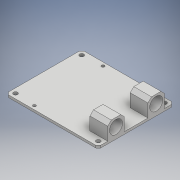
# Autodesk Inventor part: powersupplymount
Saved by Autodesk Inventor 2018.3 (Build 223284000, 284)
## iProperties
Created: 2019-05-29
Part Number: powersupplymount
Material: Generic
Document SubType Name: Modeling
Designer: matth
Density: 1 g/cm^3
Appearance: Default
Author: matth
Autodesk Inventor part; units mm, degrees
ref_plane "YZ Plane" through (0, 0, 0) normal (1, 0, 0) x (0, 1, 0)
ref_plane "XZ Plane" through (0, 0, 0) normal (0, 1, 0) x (-1, 0, 0)
ref_plane "XY Plane" through (0, 0, 0) normal (0, 0, 1) x (1, 0, 0)
sketch "Sketch1" plane through (0, 0, 0) normal (0, 0, 1) x (1, 0, 0)
  line L0 (-9.8382, 8.8164) -> (64.1618, 8.8164)
  line L1 (66.1618, 6.8164) -> (66.1618, -53.1836)
  line L2 (64.1618, -55.1836) -> (-9.8382, -55.1836)
  line L3 (-11.8382, -53.1836) -> (-11.8382, 6.8164)
  line L4 (-9.8382, 8.8164) -> (-11.8382, 6.8164)
  line L5 (64.1618, 8.8164) -> (66.1618, 6.8164)
  line L6 (66.1618, -53.1836) -> (64.1618, -55.1836)
  line L7 (-11.8382, -53.1836) -> (-9.8382, -55.1836)
  circle A0 centre (9.1618, 5.8164) radius 1.25
  circle A1 centre (9.1618, -52.1836) radius 1.25
  circle A2 centre (-7.8382, 4.8164) radius 1.75
  circle A3 centre (-7.8382, -51.1836) radius 1.75
  circle A4 centre (62.1618, -51.1836) radius 1.75
  circle A5 centre (62.1618, 4.8164) radius 1.75
  point P0 (0, 0)
  point P1 (-11.8382, 8.8164)
  point P2 (66.1618, -55.1836)
  point P3 (66.1618, 8.8164)
  point P4 (-11.8382, -55.1836)
  dimension "d0" = 78
  dimension "d1" = 64
  dimension "d2" = 2
  dimension "d3" = 2
  dimension "d4" = 2
  dimension "d5" = 2
  dimension "d6" = 2
  dimension "d7" = 2
  dimension "d8" = 2
  dimension "d9" = 2
  dimension "d10" = 2.5
  dimension "d11" = 21
  dimension "d12" = 3
  dimension "d13" = 2.5
  dimension "d14" = 3
  dimension "d15" = 21
  dimension "d16" = 3.5
  dimension "d17" = 4
  dimension "d18" = 4
  dimension "d19" = 3.5
  dimension "d20" = 4
  dimension "d21" = 4
  dimension "d22" = 3.5
  dimension "d23" = 4
  dimension "d24" = 4
  dimension "d25" = 3.5
  dimension "d26" = 4
  dimension "d27" = 4
  constraints: 16 end point, 8 point on line, 6 centre point, 2 parallel, 1 horizontal, 1 perpendicular
  measures "d0" distance of point (66.162, -55.184) point (-11.838, -55.184)
  measures "d1" distance of point (66.162, 8.816) point (66.162, -55.184)
  measures "d2" distance of L0.start point (-11.838, 8.816)
  measures "d3" distance of L3.end point (-11.838, 8.816)
  measures "d4" distance of L0.end point (66.162, 8.816)
  measures "d5" distance of L1.start point (66.162, 8.816)
  measures "d6" distance of L1.end point (66.162, -55.184)
  measures "d7" distance of L2.start point (66.162, -55.184)
  measures "d8" distance of L3.start point (-11.838, -55.184)
  measures "d9" distance of L2.end point (-11.838, -55.184)
  measures "d10" diameter of A0
  measures "d11" distance from line of L3 A0.centre
  measures "d12" distance from line of L0 A0.centre
  measures "d13" diameter of A1
  measures "d14" distance from line of L2 A1.centre
  measures "d15" distance from line of L3 A1.centre
  measures "d16" diameter of A2
  measures "d17" distance from line of L0 A2.centre
  measures "d18" distance from line of L3 A2.centre
  measures "d19" diameter of A3
  measures "d20" distance from line of L3 A3.centre
  measures "d21" distance from line of L2 A3.centre
  measures "d22" diameter of A4
  measures "d23" distance from line of L1 A4.centre
  measures "d24" distance from line of L2 A4.centre
  measures "d25" diameter of A5
  measures "d26" distance from line of L0 A5.centre
  measures "d27" distance from line of L1 A5.centre
extrude "Extrusion1" add sketch "Sketch1" along normal blind 2
sketch "Sketch2" plane through (0, 0, 2) normal (0, 0, 1) x (1, 0, 0)
  line L0 (66.1618, -53.1836) -> (66.1618, 6.8164) projected
  line L1 (66.1618, 0.8164) -> (51.1618, 0.8164)
  line L2 (51.1618, 0.8164) -> (51.1618, -13.1836)
  line L3 (51.1618, -13.1836) -> (66.1618, -13.1836)
  line L4 (66.1618, -13.1836) -> (66.1618, 0.8164)
  line L5 (64.1618, 8.8164) -> (-9.8382, 8.8164) projected
  line L6 (66.1618, -47.1836) -> (51.1618, -47.1836)
  line L7 (51.1618, -47.1836) -> (51.1618, -33.1836)
  line L8 (51.1618, -33.1836) -> (66.1618, -33.1836)
  line L9 (66.1618, -33.1836) -> (66.1618, -47.1836)
  line L10 (-9.8382, -55.1836) -> (64.1618, -55.1836) projected
  point P0 (0, 0)
  dimension "d30" = 15
  dimension "d31" = 14
  dimension "d32" = 8
  dimension "d33" = 14
  dimension "d34" = 8
  constraints: 16 end point, 4 parallel, 2 horizontal, 2 perpendicular, 2 point on line
  measures "d30" distance of L3.end L2.end
  measures "d31" distance of L1.end L2.end
  measures "d32" distance between parallel lines of L5 L1
  measures "d33" distance of L6.end L7.end
  measures "d34" distance between parallel lines of L10 L6
extrude "Extrusion2" add sketch "Sketch2" along normal blind 14
sketch "Sketch3" plane through (66.1618, -53.1836, 0) normal (1, 0, 0) x (0, 0, -1)
  circle A0 centre (-9, 13) radius 5.5
  line L0 (-2, 6) -> (-16, 6) projected
  line L1 (-16, 6) -> (-16, 20) projected
  circle A1 centre (-9, 47) radius 5.5
  line L2 (-16, 40) -> (-16, 54) projected
  line L3 (-2, 40) -> (-16, 40) projected
  point P0 (0, 53.1836)
  dimension "d37" = 11
  dimension "d38" = 7
  dimension "d39" = 7
  dimension "d40" = 11
  dimension "d41" = 7
  dimension "d42" = 7
  constraints: 2 centre point
  measures "d37" diameter of A0
  measures "d38" distance from line of L0 A0.centre
  measures "d39" distance from line of L1 A0.centre
  measures "d40" diameter of A1
  measures "d41" distance from line of L2 A1.centre
  measures "d42" distance from line of L3 A1.centre
extrude "Extrusion3" cut sketch "Sketch3" against normal up to surface (15 mm away)
chamfer "Chamfer1" distance 3 angle 45 4 edges at (58.6618, 0.8164, 16) (58.6618, -13.1836, 16) (58.6618, -33.1836, 16) (58.6618, -47.1836, 16)
equation "\"d3\" = d2"
equation "\"d4\" = d2"
equation "\"d5\" = d4"
equation "\"d6\" = d2"
equation "\"d7\" = d6"
equation "\"d8\" = d2"
equation "\"d9\" = d8"
body "Solid1"
